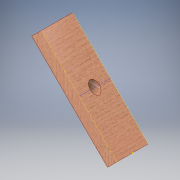
# Autodesk Inventor part: 2x4x12
Saved by Autodesk Inventor 2019.4 (Build 234330000, 330)
## iProperties
Created: 2019-06-16
Part Number: 2x4x12
Material: Wood (Oak)
Document SubType Name: Modeling
Designer: steele
Density: 0.76 g/cm^3
Appearance: White Oak - Natural Medium Gloss
Author: steele
Autodesk Inventor part; units mm, degrees
ref_plane "YZ Plane" through (0, 0, 0) normal (1, 0, 0) x (0, 1, 0)
ref_plane "XY Plane" through (0, 0, 0) normal (0, 0, 1) x (1, 0, 0)
sketch "Sketch1" plane through (0, 0, 0) normal (0, 0, 1) x (1, 0, 0)
  line L0 (0, 0) -> (-215.5261, 215.5261)
  line L1 (0, 0) -> (304.8, 0) construction
  line L2 (-215.5261, 215.5261) -> (-188.5854, 242.4669)
  line L3 (-215.5261, 215.5261) -> (-177.4261, 215.5261) construction
  line L4 (0, 0) -> (26.9408, 26.9408)
  line L5 (0, 0) -> (38.1, 0) construction
  line L6 (26.9408, 26.9408) -> (-188.5854, 242.4669)
  dimension "boardLength" = 304.8
  dimension "d1" = 135
  dimension "boardDepth" = 38.1
  dimension "d3" = 45
  dimension "d4" = 38.1
  dimension "d5" = 45
  constraints: 14 end point, 3 equal length, 3 horizontal, 1 perpendicular
  measures "boardLength" distance of L0.start L0.end
  measures "d1" angle of L1 L0
  measures "boardDepth" distance of L0.end L2.end
  measures "d3" angle of L3 L2
  measures "d4" distance of L0.start L4.end
  measures "d5" angle of L5 L4
extrude "Extrusion1" add sketch "Sketch1" along normal mid plane 88.9
sketch "Sketch3" plane through (-188.5854, 242.4669, -44.45) normal (0.7071, 0.7071, 0) x (-0.7071, 0.7071, 0)
  line L0 (0, 88.9) -> (-304.8, 88.9) construction
  line L1 (-152.4, 88.9) -> (-152.4, 0) construction
  line L2 (0, 0) -> (-304.8, 0) construction
  point P0 (-304.8, 44.45)
  constraints: 2 end point, 2 midpoint
ref_plane "Work Plane1" through (-80.8223, 134.7038, 44.45) normal (1, 0, 0) x (0, 0, -1)
sketch "Sketch4" plane through (-80.8223, 134.7038, 44.45) normal (1, 0, 0) x (0, 0, -1)
  line L0 (0, -107.7631) -> (0, 107.7631) projected
  circle A0 centre (44.45, 0) radius 12.7
  point P0 (44.45, -134.7038)
  dimension "d17" = 25.4
  constraints: 1 centre point
  measures "d17" diameter of A0
extrude "Extrusion2" cut sketch "Sketch4" along normal through all both and the other way through all
equation "\"d4\" = boardDepth"
body "Solid1"
